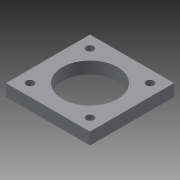
# Autodesk Inventor part: BallBearingHolderOutside
Saved by Autodesk Inventor 2015 (Build 190159000, 159)
## iProperties
Created: 2017-03-08
Part Number: BallBearingHolderOutside
Material: Generic
Document SubType Name: Modeling
Designer: Ernest
Density: 1 g/cm^3
Appearance: Default
Author: Ernest
Autodesk Inventor part; units mm, degrees
ref_plane "YZ Plane" through (0, 0, 0) normal (1, 0, 0) x (0, 1, 0)
ref_plane "XZ Plane" through (0, 0, 0) normal (0, 1, 0) x (-1, 0, 0)
ref_plane "XY Plane" through (0, 0, 0) normal (0, 0, 1) x (1, 0, 0)
sketch "Sketch1" plane through (0, 0, 0) normal (0, 0, 1) x (1, 0, 0)
  circle A0 centre (0, 0) radius 11.5
  circle A1 centre (0, 0) radius 14.3 construction
  line L0 (-17.5, 17.5) -> (17.5, 17.5)
  line L1 (17.5, 17.5) -> (17.5, -17.5)
  line L2 (17.5, -17.5) -> (-17.5, -17.5)
  line L3 (-17.5, -17.5) -> (-17.5, 17.5)
  line L4 (-12.5, 12.5) -> (12.5, 12.5) construction
  line L5 (12.5, 12.5) -> (12.5, -12.5) construction
  line L6 (12.5, -12.5) -> (-12.5, -12.5) construction
  line L7 (-12.5, -12.5) -> (-12.5, 12.5) construction
  line L8 (-10.0913, 14.9087) -> (-9.2097, 11.6184)
  line L9 (-9.2097, 11.6184) -> (-11.6184, 9.2097)
  line L10 (-11.6184, 9.2097) -> (-14.9087, 10.0913)
  line L11 (-14.9087, 10.0913) -> (-15.7903, 13.3816)
  line L12 (-15.7903, 13.3816) -> (-13.3816, 15.7903)
  line L13 (-13.3816, 15.7903) -> (-10.0913, 14.9087)
  line L14 (14.9087, 10.0913) -> (11.6184, 9.2097)
  line L15 (11.6184, 9.2097) -> (9.2097, 11.6184)
  line L16 (9.2097, 11.6184) -> (10.0913, 14.9087)
  line L17 (10.0913, 14.9087) -> (13.3816, 15.7903)
  line L18 (13.3816, 15.7903) -> (15.7903, 13.3816)
  line L19 (15.7903, 13.3816) -> (14.9087, 10.0913)
  line L20 (14.9087, -10.0913) -> (15.7903, -13.3816)
  line L21 (15.7903, -13.3816) -> (13.3816, -15.7903)
  line L22 (13.3816, -15.7903) -> (10.0913, -14.9087)
  line L23 (10.0913, -14.9087) -> (9.2097, -11.6184)
  line L24 (9.2097, -11.6184) -> (11.6184, -9.2097)
  line L25 (11.6184, -9.2097) -> (14.9087, -10.0913)
  line L26 (-14.9087, -10.0913) -> (-11.6184, -9.2097)
  line L27 (-11.6184, -9.2097) -> (-9.2097, -11.6184)
  line L28 (-9.2097, -11.6184) -> (-10.0913, -14.9087)
  line L29 (-10.0913, -14.9087) -> (-13.3816, -15.7903)
  line L30 (-13.3816, -15.7903) -> (-15.7903, -13.3816)
  line L31 (-15.7903, -13.3816) -> (-14.9087, -10.0913)
  line L32 (-12.5, 12.5) -> (12.5, -12.5) construction
  line L33 (12.5, 12.5) -> (-12.5, -12.5) construction
  circle A2 centre (-12.5, 12.5) radius 1.6
  circle A3 centre (12.5, 12.5) radius 1.6
  circle A4 centre (12.5, -12.5) radius 1.6
  circle A5 centre (-12.5, -12.5) radius 1.6
  dimension "d0" = 28.6
  dimension "d1" = 23
  dimension "d6" = 5.9
  dimension "d7" = 25
  dimension "d8" = 25
  dimension "d9" = 3.2
  dimension "d10" = 35
  dimension "d11" = 17.5
  dimension "d12" = 35
  dimension "d13" = 17.5
  constraints: 68 end point, 10 coincident, 6 centre point, 6 perpendicular, 4 parallel, 3 equal length, 3 equal radius, 2 horizontal, 2 midpoint, 52 other
  measures "d0" diameter of A1
  measures "d1" diameter of A0
  measures "d6" distance between parallel lines of L10 L13
  measures "d7" distance of L4.start L4.end
  measures "d8" distance of L6.end L4.start
  measures "d9" diameter of A2
  measures "d10" distance of L1.end L2.end
  measures "d11" distance from line of point (0, 0) L3
  measures "d12" distance of L0.end L1.end
  measures "d13" distance from line of point (0, 0) L0
extrude "Extrusion3" add sketch "Sketch1" along normal blind 5 contours L0 L1 L2 L3 | L8 L9 L10 L11 L12 L13 | L14 L15 L16 L17 L18 L19 | L20 L21 L22 L23 L24 L25 | L26 L27 L28 L29 L30 L31
extrude "Extrusion4" cut sketch "Sketch1" along normal blind 2.3 contours L8 L9 L10 L11 L12 L13 | L14 L15 L16 L17 L18 L19 | L20 L21 L22 L23 L24 L25 | L26 L27 L28 L29 L30 L31
equation "\"d11\" = 0.5 * d10"
equation "\"d13\" = 0.5 * d12"
body "Solid2"
